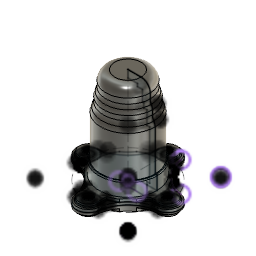
hw3 (Autodesk Fusion 360 design; units mm, degrees)
part number: 2026-08-06-11-14-22-683
Autodesk Fusion 360 part; units mm, degrees
sketch "스케치1" plane through (0, 0, 0) normal (0, 0, 1) x (1, 0, 0)
  circle A0 centre (0, 0) radius 44 construction
  arc A1 (12.8574, 42.0795) -> (-12.8574, 42.0795) centre (0, 44) ccw
  arc A2 (-42.0795, 12.8574) -> (-42.0795, -12.8574) centre (-44, 0) ccw
  arc A3 (-12.8574, -42.0795) -> (12.8574, -42.0795) centre (0, -44) ccw
  arc A4 (42.0795, -12.8574) -> (42.0795, 12.8574) centre (44, 0) ccw
  arc A5 (12.8655, 45.8655) -> (45.8655, 12.8655) centre (51.4618, 51.4618) ccw
  arc A6 (-45.8655, 12.8655) -> (-12.8655, 45.8655) centre (-51.4618, 51.4618) ccw
  arc A7 (-12.8655, -45.8655) -> (-45.8655, -12.8655) centre (-51.4618, -51.4618) ccw
  arc A8 (45.8655, -12.8655) -> (12.8655, -45.8655) centre (51.4618, -51.4618) ccw
  dimension "d1" = 88
  dimension "d2" = 26
  dimension "d3" = 44
  dimension "d5" = 360
  dimension "d20" = 78
  dimension "d22" = 360
  constraint coincident A0.centre origin
  constraint coincident A0 A1.centre
  constraint coincident A0 A1.end
  constraint coincident A0 A1.start
  constraint coincident A0 A2.end
  constraint coincident A0 A2.start
  constraint coincident A0 A3.end
  constraint coincident A0 A3.start
  constraint coincident A0 A4.end
  constraint coincident A0 A4.start
  constraint tangent A1 A5
  constraint tangent A4 A5
  constraint coincident A4 A5.end
  constraint coincident A1 A5.start
  measures "d1" diameter of A0
  measures "d2" diameter of A1
  measures "d3" vertical distance of A0.centre A1.centre
  measures "d20" diameter of A5
extrude "돌출1" add sketch "스케치1" along normal blind 3
ref_plane "작업 평면1" through (0, 0, 3) normal (0, 0, 1) x (1, 0, 0)
sketch "스케치2" plane through (0, 0, 3) normal (0, 0, 1) x (1, 0, 0)
  line L0 (0, 0) -> (0, 44) construction
  circle A0 centre (0, 44) radius 10
  circle A1 centre (0, 44) radius 5
  circle A2 centre (-44, 0) radius 5
  circle A3 centre (-44, 0) radius 10
  circle A4 centre (0, -44) radius 5
  circle A5 centre (0, -44) radius 10
  circle A6 centre (44, 0) radius 5
  circle A7 centre (44, 0) radius 10
  line L1 (10, 44) -> (10, 33.541)
  line L2 (44, 10) -> (33.541, 10)
  line L3 (-44, 10) -> (-33.541, 10)
  line L4 (-10, 44) -> (-10, 33.541)
  line L5 (-10, -44) -> (-10, -33.541)
  line L6 (-44, -10) -> (-33.541, -10)
  line L7 (44, -10) -> (33.541, -10)
  line L8 (10, -44) -> (10, -33.541)
  arc A8 (-13.125, 32.4459) -> (-10, 37.081) centre (-15, 37.081) ccw
  arc A9 (10, 37.081) -> (13.125, 32.4459) centre (15, 37.081) ccw
  arc A10 (32.4459, 13.125) -> (37.081, 10) centre (37.081, 15) ccw
  arc A11 (37.081, -10) -> (32.4459, -13.125) centre (37.081, -15) ccw
  arc A12 (13.125, -32.4459) -> (10, -37.081) centre (15, -37.081) ccw
  arc A13 (-10, -37.081) -> (-13.125, -32.4459) centre (-15, -37.081) ccw
  arc A14 (-37.081, 10) -> (-32.4459, 13.125) centre (-37.081, 15) ccw
  arc A15 (-32.4459, -13.125) -> (-37.081, -10) centre (-37.081, -15) ccw
  line L9 (-37.081, 15) -> (-37.081, -15) construction
  arc A16 (12.8655, 45.8655) -> (45.8655, 12.8655) centre (51.4618, 51.4618) ccw
  arc A17 (19.5652, 29.0208) -> (-19.5652, 29.0208) centre (0, 0) ccw
  arc A18 (-29.0208, 19.5652) -> (-29.0208, -19.5652) centre (0, 0) ccw
  arc A19 (-19.5652, -29.0208) -> (19.5652, -29.0208) centre (0, 0) ccw
  arc A20 (29.0208, -19.5652) -> (29.0208, 19.5652) centre (0, 0) ccw
  arc A21 (-29.0208, 19.5652) -> (-19.5652, 29.0208) centre (-51.4618, 51.4618) ccw
  arc A22 (-19.5652, -29.0208) -> (-29.0208, -19.5652) centre (-51.4618, -51.4618) ccw
  arc A23 (29.0208, -19.5652) -> (19.5652, -29.0208) centre (51.4618, -51.4618) ccw
  arc A24 (19.5652, 29.0208) -> (29.0208, 19.5652) centre (51.4618, 51.4618) ccw
  point P0 (-44, 0)
  point P1 (0, -44)
  point P2 (44, 0)
  point P3 (51.4618, 51.4618)
  point P4 (51.4618, -51.4618)
  dimension "d13" = 44
  dimension "d14" = 20
  dimension "d15" = 10
  dimension "d17" = 360
  dimension "d18" = 10
  dimension "d19" = 70
  dimension "d23" = 10
  dimension "d25" = 360
  dimension "d27" = 78
  dimension "d29" = 360
  constraint coincident L0.start A17.centre
  constraint vertical L0
  constraint coincident L0.end A0.centre
  constraint concentric A0 A1
  constraint vertical L1
  constraint tangent A0 L1
  constraint tangent L1 A9
  constraint tangent A9 A17
  constraint perpendicular L0 L2
  constraint tangent A7 L2
  constraint tangent L2 A10
  constraint tangent A10 A20
  constraint coincident A0 L1.start
  constraint coincident L1.end A17
  constraint coincident L2.end A20
  constraint coincident A7 L2.start
  constraint coincident L4 A8.end
  constraint coincident A8.start A17
  constraint coincident A9.end A17
  constraint coincident L1 A9.start
  constraint coincident L2 A10.end
  constraint coincident A10.start A20
  constraint coincident A11.end A20
  constraint coincident L7 A11.start
  constraint coincident L8 A12.end
  constraint coincident A12.start A19
  constraint coincident A13.end A19
  constraint coincident L5 A13.start
  constraint coincident A14.end A18
  constraint coincident L3 A14.start
  constraint coincident L6 A15.end
  constraint coincident A15.start A18
  constraint coincident A14.centre L9.start
  constraint coincident A15.centre L9.end
  constraint coincident A17.start A16
  constraint coincident A20.end A16
  constraint coincident P4 A23.centre
  constraint concentric A17 A18
  constraint concentric A18 A19
  constraint concentric A19 A20
  measures "d13" distance of L0.start L0.end
  measures "d14" diameter of A0
  measures "d15" diameter of A1
  measures "d18" diameter of A9
  measures "d19" diameter of A17
  measures "d23" diameter of A10
  measures "d27" diameter of A23
extrude "돌출2" add sketch "스케치2" along normal blind 3 contours A0 A17 | A0 L1 A17 | A0 L4 A17 | A0 A3 A5 A7 A16 A17 A18 A19 A20 A21 A22 A23 A24 | A0 A17 | L1 A9 A17 | L4 A8 A17 | L2 A10 A20 | L3 A14 A18 | A7 L2 A20 | A3 L3 A18 | A7 A20 | A7 A20 | A3 A18 | A3 A18 | A7 L7 A20 | A3 L6 A18 | L7 A11 A20 | L6 A15 A18 | L5 A13 A19 | A5 L8 A19 | A5 L5 A19 | A5 A19 | A5 A19
extrude "돌출3" cut sketch "스케치2" against normal blind 6 contours A1 | A2 | A4 | A6
mirror "미러1" about plane through (0, 0, 0) normal (0, 0, 1) of bodies 1 merged
sketch "스케치3" plane through (0, 0, 0) normal (0, 1, 0) x (1, 0, 0)
  line L0 (0, 6) -> (0, -106) construction
  line L1 (-10, 6) -> (10, 6)
  line L2 (0, -106) -> (14.5, -106)
  line L3 (24.5, -96) -> (24.5, -90.1515)
  arc A0 (14.5, -106) -> (24.5, -96) centre (14.5, -96) ccw
  line L4 (24, -9) -> (24, -63)
  line L5 (21, -63) -> (21, -78)
  line L6 (21, -63) -> (24, -63)
  line L7 (17.5, -78) -> (17.5, -83)
  line L8 (17.5, -78) -> (21, -78)
  line L9 (16, -83) -> (16, -95)
  line L10 (16, -83) -> (17.5, -83)
  line L11 (10.5, -95) -> (10.5, -98)
  line L12 (16, -95) -> (10.5, -95)
  line L13 (10.5, -98) -> (0, -98)
  line L14 (32, -6) -> (32, -21)
  line L15 (21, -6) -> (0, -6)
  line L16 (0, -6) -> (0, 6)
  line L17 (0, 6) -> (21, 6)
  line L18 (21, 6) -> (21, -6)
  line L19 (21, -9) -> (21, 6)
  line L20 (21, -9) -> (24, -9)
  line L21 (30, -21) -> (30, -66)
  line L22 (30, -21) -> (32, -21)
  line L23 (27, -81) -> (27, -75.9499)
  arc A1 (25.75, -85.5758) -> (24.5, -90.1515) centre (33.5, -90.1515) ccw
  arc A2 (28.5, -70.9749) -> (27, -75.9499) centre (36, -75.9499) ccw
  arc A3 (25.75, -85.5758) -> (27, -81) centre (18, -81) ccw
  arc A4 (28.5, -70.9749) -> (30, -66) centre (21, -66) ccw
  line L24 (32, -6) -> (21, -6)
  line L25 (0, -98) -> (0, -106)
  dimension "d38" = 112
  dimension "d40" = 24.5
  dimension "d41" = 20
  dimension "d45" = 24
  dimension "d46" = 15
  dimension "d47" = 21
  dimension "d48" = 5
  dimension "d49" = 17.5
  dimension "d50" = 12
  dimension "d51" = 16
  dimension "d52" = 3
  dimension "d53" = 10.5
  dimension "d54" = 32
  dimension "d56" = 12
  dimension "d58" = 21
  dimension "d59" = 15
  dimension "d60" = 54
  dimension "d61" = 6
  dimension "d62" = 27
  dimension "d63" = 30
  dimension "d65" = 40
  dimension "d67" = 25
  dimension "d70" = 27
  dimension "d71" = 9
  dimension "d72" = 9
  dimension "d73" = 9
  dimension "d74" = 9
  constraint vertical L0
  constraint coincident L0.start L1
  constraint coincident L0 origin
  constraint perpendicular L0 L2
  constraint vertical L3
  constraint tangent L2 A0
  constraint tangent L3 A0
  constraint parallel L4 L5
  constraint perpendicular L4 L6
  constraint parallel L5 L7
  constraint perpendicular L5 L8
  constraint parallel L7 L9
  constraint perpendicular L7 L10
  constraint parallel L9 L11
  constraint perpendicular L11 L12
  constraint coincident L0 L13.end
  constraint perpendicular L0 L13
  constraint vertical L14
  constraint horizontal L15
  constraint vertical L16
  constraint horizontal L17
  constraint vertical L18
  constraint perpendicular L17 L19
  constraint perpendicular L19 L20
  constraint parallel L14 L21
  constraint tangent L21 A4
  constraint perpendicular L14 L22
  constraint tangent L3 A1
  constraint tangent A1 A3
  constraint vertical L23
  constraint tangent A2 A4
  constraint tangent L23 A2
  constraint tangent L23 A3
  measures "d38" distance of L0.start L0.end
  measures "d40" distance of L0 L3
  measures "d41" diameter of A0
  measures "d45" distance of L0 L4
  measures "d46" distance of L5.start L5.end
  measures "d47" distance of L0 L5
  measures "d48" distance of L7.start L7.end
  measures "d49" distance of L0 L7
  measures "d50" distance of L9.start L9.end
  measures "d51" distance of L0 L9
  measures "d52" distance of L11.start L11.end
  measures "d53" distance of L0 L11
  measures "d54" distance of L0 L14.start
  measures "d56" distance of L15.start L17.end
  measures "d58" distance of L0 L19
  measures "d59" distance of L19.start L17.end
  measures "d60" distance of L6 L20
  measures "d61" vertical distance of origin L14.start
  measures "d62" vertical distance of L0.start L14.end
  measures "d63" distance of L0 L21
  measures "d65" distance of L2 A4.centre
  measures "d67" distance of L2 A3.centre
  measures "d70" distance of L0 L23
  measures "d71" radius of A4
  measures "d72" radius of A2
  measures "d73" radius of A3
  measures "d74" radius of A1
revolve "회전1" cut sketch "스케치3" angle 360 about axis through (0, 0, -6) along (0, 0, 1) contours L1 L15 L16 L17 L18 L19
revolve "회전2" add sketch "스케치3" angle 360 about axis through (0, 0, -6) along (0, 0, 1) contours L2 L3 A0 L4 L5 L6 L7 L8 L9 L10 L11 L12 L13 L14 L19 L20 L21 L22 L23 A1 A2 A3 A4 L24 L25
fillet "필렛1" radius 1 5 edges at (10, -38.7705, 3) (0, -54, 3) (-10, -40.5405, 3) (-10.8542, -34.2859, 3) (-16.4346, -30.9015, 3)
fillet "필렛2" radius 1 7 edges at (-30.9015, -16.4346, 3) (-34.2859, -10.8542, 3) (-40.5405, -10, 3) (-54, 0, 3) (-40.5405, 10, 3) (-34.2859, 10.8542, 3) (-30.9015, 16.4346, 3)
fillet "필렛3" radius 1 7 edges at (-16.4346, 30.9015, 3) (-10.8542, 34.2859, 3) (-10, 40.5405, 3) (0, 54, 3) (10, 40.5405, 3) (10.8542, 34.2859, 3) (16.4346, 30.9015, 3)
fillet "필렛4" radius 1 7 edges at (30.9015, 16.4346, 3) (34.2859, 10.8542, 3) (40.5405, 10, 3) (54, 0, 3) (40.5405, -10, 3) (34.2859, -10.8542, 3) (30.9015, -16.4346, 3)
fillet "필렛5" radius 1 22 edges at (-30.9015, -16.4346, -3) (-34.2859, -10.8542, -3) (-40.5405, -10, -3) (-54, 0, -3) (-40.5405, 10, -3) (-34.2859, 10.8542, -3) (-30.9015, 16.4346, -3) (-16.4346, 30.9015, -3) (-10.8542, 34.2859, -3) (-10, 40.5405, -3) (0, 54, -3) (10, 40.5405, -3) (10.8542, 34.2859, -3) (16.4346, 30.9015, -3) (10, -38.7705, -3) (0, -54, -3) (-10, -40.5405, -3) (-10.8542, -34.2859, -3) (-16.4346, -30.9015, -3) (37.0484, -15.223, -3) (57, 0, -3) (37.0484, 15.223, -3)
fillet "필렛6" radius 0.5 1 edges at (-9.7894, -3.797, 95)
fillet "필렛7" radius 0.5 3 edges at (-14.9172, -5.7858, 83) (-16.3157, -6.3283, 78) (-19.5789, -7.5939, -6)
fillet "필렛8" radius 1 1 edges at (-29.8345, -11.5717, 21)
